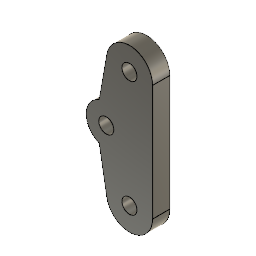
x_idler (Autodesk Fusion 360 design; units mm, degrees)
Autodesk Fusion 360 part; units mm, degrees
note: some values were not read from the file. Set by a fixed rule: which sketch regions a step uses.
sketch "Sketch1" plane through (0, 0, 0) normal (0, 1, 0) x (1, 0, 0)
  line L0 (0, 0) -> (0, -20) construction
  circle A0 centre (0, 0) radius 2.6
  circle A1 centre (8, -20) radius 2.6
  line L1 (0, -20) -> (8, -20) construction
  line L2 (0, 0) -> (18.1281, 0) construction
  circle A2 centre (8, 20) radius 2.6
  circle A3 centre (8, 20) radius 8
  circle A4 centre (0, 0) radius 7
  circle A5 centre (8, -20) radius 8
  line L3 (16, 20) -> (16, -20)
  line L4 (0.4465, 22.6352) -> (0.4465, 23.2319)
  line L5 (0.4465, 23.2319) -> (-2.4969, 6.5396)
  line L6 (0.4465, -23.2319) -> (-2.4969, -6.5396)
  dimension "d1" = 5.2
  dimension "d2" = 8
  dimension "d3" = 20
  dimension "d4" = 16
  dimension "d5" = 14
  dimension "d8" = 10
  measures "d1" diameter of A0
  measures "d2" distance of L0.start
  measures "d4" diameter of A3
  measures "d5" diameter of A4
  measures "d8" angle of L0 L5
extrude "Extrude1" add sketch "Sketch1" along normal blind 6 contours A3 | A3 A4 A5 L3 L5 L6 | A5 | A4
